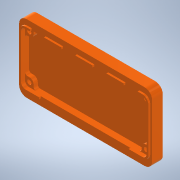
# Autodesk Inventor part: casing-bot
Saved by Autodesk Inventor 2021 (Build 250183000, 183)
## iProperties
Created: 2022-04-04
Part Number: casing-bot
Material: PET Plastic
Document SubType Name: Modeling
Designer: Staňa
Density: 1.541 g/cm^3
Appearance: Smooth - Light Orange
Author: Staňa
Autodesk Inventor part; units mm, degrees
ref_plane "YZ Plane" through (0, 0, 0) normal (1, 0, 0) x (0, 1, 0)
ref_plane "XZ Plane" through (0, 0, 0) normal (0, 1, 0) x (-1, 0, 0)
ref_plane "XY Plane" through (0, 0, 0) normal (0, 0, 1) x (1, 0, 0)
sketch "Sketch2" plane through (0, 0, 0) normal (0, 0, 1) x (1, 0, 0)
  line L0 (-50, -20) -> (-50, 15) construction
  arc A0 (-46.75, 18.25) -> (-50, 15) centre (-46.7497, 14.9997) ccw construction
  line L1 (-46.75, 18.25) -> (46.75, 18.25) construction
  arc A1 (50, 15) -> (46.75, 18.25) centre (46.7497, 14.9997) ccw construction
  line L2 (50, 15) -> (50, -20) construction
  arc A2 (46.75, -23.25) -> (50, -20) centre (46.7497, -19.9997) ccw construction
  line L3 (46.75, -23.25) -> (-46.75, -23.25) construction
  arc A3 (-50, -20) -> (-46.75, -23.25) centre (-46.7497, -19.9997) ccw construction
  circle A4 centre (-46.75, -22.184) radius 0.254 construction
  circle A5 centre (-48.934, -20) radius 0.254 construction
  circle A6 centre (-48.295, -21.545) radius 0.254 construction
  circle A7 centre (-45.205, -21.545) radius 0.254 construction
  circle A8 centre (-27.94, -19.9) radius 0.51 construction
  circle A9 centre (-44.566, -20) radius 0.254 construction
  circle A10 centre (-25.4, -19.9) radius 0.51 construction
  circle A11 centre (-48.295, -18.455) radius 0.254 construction
  circle A12 centre (-46.75, -20) radius 1.6 construction
  circle A13 centre (-46.75, -17.816) radius 0.254 construction
  circle A14 centre (-45.205, -18.455) radius 0.254 construction
  circle A15 centre (-30.48, -17.36) radius 0.51 construction
  circle A16 centre (-30.48, -19.9) radius 0.51 construction
  circle A17 centre (-27.94, -17.36) radius 0.51 construction
  circle A18 centre (-25.4, -17.36) radius 0.51 construction
  circle A19 centre (-17.78, -19.9) radius 0.51 construction
  circle A20 centre (-22.86, -19.9) radius 0.51 construction
  circle A21 centre (-20.32, -19.9) radius 0.51 construction
  circle A22 centre (-10.16, -19.9) radius 0.51 construction
  circle A23 centre (-7.62, -19.9) radius 0.51 construction
  circle A24 centre (-15.24, -19.9) radius 0.51 construction
  circle A25 centre (-12.7, -19.9) radius 0.51 construction
  circle A26 centre (-12.7, -17.36) radius 0.51 construction
  circle A27 centre (-5.08, -19.9) radius 0.51 construction
  circle A28 centre (-7.62, -17.36) radius 0.51 construction
  circle A29 centre (-5.08, -17.36) radius 0.51 construction
  circle A30 centre (-2.54, -19.9) radius 0.51 construction
  circle A31 centre (0, -19.9) radius 0.51 construction
  circle A32 centre (-2.54, -17.36) radius 0.51 construction
  circle A33 centre (0, -17.36) radius 0.51 construction
  circle A34 centre (-46.75, 12.816) radius 0.254 construction
  circle A35 centre (-48.295, 13.455) radius 0.254 construction
  circle A36 centre (-45.205, 13.455) radius 0.254 construction
  circle A37 centre (-41.31, 11.85) radius 0.51 construction
  circle A38 centre (-38.77, 11.85) radius 0.51 construction
  circle A39 centre (-41.31, 14.39) radius 0.51 construction
  circle A40 centre (-36.23, 11.85) radius 0.51 construction
  circle A41 centre (-48.934, 15) radius 0.254 construction
  circle A42 centre (-46.75, 15) radius 1.6 construction
  circle A43 centre (-48.295, 16.545) radius 0.254 construction
  circle A44 centre (-46.75, 17.184) radius 0.254 construction
  circle A45 centre (-38.77, 14.39) radius 0.51 construction
  circle A46 centre (-36.23, 14.39) radius 0.51 construction
  circle A47 centre (-45.205, 16.545) radius 0.254 construction
  circle A48 centre (-44.566, 15) radius 0.254 construction
  circle A49 centre (-20.32, -17.36) radius 0.51 construction
  circle A50 centre (-33.69, 11.85) radius 0.51 construction
  circle A51 centre (-22.86, -17.36) radius 0.51 construction
  circle A52 centre (-17.78, -17.36) radius 0.51 construction
  circle A53 centre (-15.24, -17.36) radius 0.51 construction
  circle A54 centre (-16.31, 11.85) radius 0.51 construction
  circle A55 centre (-10.16, -17.36) radius 0.51 construction
  circle A56 centre (-16.31, 14.39) radius 0.51 construction
  circle A57 centre (-13.77, 11.85) radius 0.51 construction
  circle A58 centre (-33.69, 14.39) radius 0.51 construction
  circle A59 centre (-13.77, 14.39) radius 0.51 construction
  circle A60 centre (-11.23, 11.85) radius 0.51 construction
  circle A61 centre (-8.69, 11.85) radius 0.51 construction
  circle A62 centre (-11.23, 14.39) radius 0.51 construction
  circle A63 centre (-8.69, 14.39) radius 0.51 construction
  circle A64 centre (10.16, -19.9) radius 0.51 construction
  circle A65 centre (5.08, -19.9) radius 0.51 construction
  circle A66 centre (7.62, -19.9) radius 0.51 construction
  circle A67 centre (20.32, -19.9) radius 0.51 construction
  circle A68 centre (22.86, -19.9) radius 0.51 construction
  circle A69 centre (12.7, -19.9) radius 0.51 construction
  circle A70 centre (15.24, -19.9) radius 0.51 construction
  circle A71 centre (2.54, -19.9) radius 0.51 construction
  circle A72 centre (7.62, -17.36) radius 0.51 construction
  circle A73 centre (10.16, -17.36) radius 0.51 construction
  circle A74 centre (12.7, -17.36) radius 0.51 construction
  circle A75 centre (15.24, -17.36) radius 0.51 construction
  circle A76 centre (17.78, -19.9) radius 0.51 construction
  circle A77 centre (17.78, -17.36) radius 0.51 construction
  circle A78 centre (20.32, -17.36) radius 0.51 construction
  circle A79 centre (25.4, -19.9) radius 0.51 construction
  circle A80 centre (30.48, -19.9) radius 0.51 construction
  circle A81 centre (44.566, -20) radius 0.254 construction
  circle A82 centre (45.205, -21.545) radius 0.254 construction
  circle A83 centre (46.75, -22.184) radius 0.254 construction
  circle A84 centre (48.295, -21.545) radius 0.254 construction
  circle A85 centre (48.934, -20) radius 0.254 construction
  circle A86 centre (22.86, -17.36) radius 0.51 construction
  circle A87 centre (27.94, -19.9) radius 0.51 construction
  circle A88 centre (25.4, -17.36) radius 0.51 construction
  circle A89 centre (27.94, -17.36) radius 0.51 construction
  circle A90 centre (45.205, -18.455) radius 0.254 construction
  circle A91 centre (46.75, -20) radius 1.6 construction
  circle A92 centre (46.75, -17.816) radius 0.254 construction
  circle A93 centre (48.295, -18.455) radius 0.254 construction
  circle A94 centre (2.54, -17.36) radius 0.51 construction
  circle A95 centre (0, 6.27) radius 0.5 construction
  circle A96 centre (0, 3.73) radius 0.5 construction
  circle A97 centre (5.08, -17.36) radius 0.51 construction
  circle A98 centre (30.48, -17.36) radius 0.51 construction
  circle A99 centre (8.69, 11.85) radius 0.51 construction
  circle A100 centre (11.23, 11.85) radius 0.51 construction
  circle A101 centre (8.69, 14.39) radius 0.51 construction
  circle A102 centre (13.77, 11.85) radius 0.51 construction
  circle A103 centre (11.23, 14.39) radius 0.51 construction
  circle A104 centre (13.77, 14.39) radius 0.51 construction
  circle A105 centre (16.31, 11.85) radius 0.51 construction
  circle A106 centre (33.69, 11.85) radius 0.51 construction
  circle A107 centre (16.31, 14.39) radius 0.51 construction
  circle A108 centre (33.69, 14.39) radius 0.51 construction
  circle A109 centre (36.23, 11.85) radius 0.51 construction
  circle A110 centre (38.77, 11.85) radius 0.51 construction
  circle A111 centre (41.31, 14.39) radius 0.51 construction
  circle A112 centre (41.31, 11.85) radius 0.51 construction
  circle A113 centre (46.75, 12.816) radius 0.254 construction
  circle A114 centre (45.205, 13.455) radius 0.254 construction
  circle A115 centre (48.295, 13.455) radius 0.254 construction
  circle A116 centre (36.23, 14.39) radius 0.51 construction
  circle A117 centre (38.77, 14.39) radius 0.51 construction
  circle A118 centre (44.566, 15) radius 0.254 construction
  circle A119 centre (45.205, 16.545) radius 0.254 construction
  circle A120 centre (46.75, 15) radius 1.6 construction
  circle A121 centre (48.934, 15) radius 0.254 construction
  circle A122 centre (46.75, 17.184) radius 0.254 construction
  circle A123 centre (48.295, 16.545) radius 0.254 construction
  line L4 (-46.7497, -23.5) -> (46.7497, -23.5)
  arc A124 (46.7497, -23.5) -> (50.25, -19.9997) centre (46.7497, -19.9997) ccw
  line L5 (50.25, -19.9997) -> (50.25, 14.9997)
  arc A125 (50.25, 14.9997) -> (46.7497, 18.5) centre (46.7497, 14.9997) ccw
  line L6 (46.7497, 18.5) -> (-46.7497, 18.5)
  arc A126 (-46.7497, 18.5) -> (-50.25, 14.9997) centre (-46.7497, 14.9997) ccw
  line L7 (-50.25, 14.9997) -> (-50.25, -19.9997)
  arc A127 (-50.25, -19.9997) -> (-46.7497, -23.5) centre (-46.7497, -19.9997) ccw
  line L8 (-32.1701, 24.2499) -> (-42.8301, 24.2499) construction
  line L9 (34.9801, -30.2999) -> (-34.9799, -30.2999) construction
  line L10 (-53.25, 18.2499) -> (-53.25, -24.2999)
  line L11 (53.25, -24.2999) -> (53.25, 18.2499)
  line L12 (-47.25, -30.2999) -> (47.25, -30.2999)
  line L13 (47.25, 24.2499) -> (-47.25, 24.2499)
  arc A128 (-53.25, -24.2999) -> (-47.25, -30.2999) centre (-47.25, -24.2999) ccw
  arc A129 (-47.25, 24.2499) -> (-53.25, 18.2499) centre (-47.25, 18.2499) ccw
  arc A130 (53.25, 18.2499) -> (47.25, 24.2499) centre (47.25, 18.2499) ccw
  arc A131 (47.25, -30.2999) -> (53.25, -24.2999) centre (47.25, -24.2999) ccw
  point P0 (0, 0)
  dimension "d4" = 0.25
  dimension "d7" = 3
  dimension "d8" = 3
  dimension "d10" = 6
  constraints: 16 end point, 16 point on circle, 8 centre point, 8 tangent, 3 equal radius, 2 collinear, 2 parallel, 7 other
  measures "d4" radial gap between concentric circles of A3 A127
  measures "d7" distance between parallel lines of L7 L10
  measures "d8" distance between parallel lines of L5 L11
  measures "d10" radius of A128
extrude "Extrusion1" add sketch "Sketch2" against normal blind 5
sketch "Sketch6" plane through (0, 0, 0) normal (0, 0, 1) x (1, 0, 0)
  line L0 (-50.25, -19.9997) -> (-50.25, 14.9997) projected
  arc A0 (-50.25, -19.9997) -> (-46.7497, -23.5) centre (-46.7497, -19.9997) ccw projected
  line L1 (46.7497, -23.5) -> (-46.7497, -23.5) projected
  arc A1 (46.7497, -23.5) -> (50.25, -19.9997) centre (46.7497, -19.9997) ccw projected
  line L2 (50.25, 14.9997) -> (50.25, -19.9997) projected
  arc A2 (50.25, 14.9997) -> (46.7497, 18.5) centre (46.7497, 14.9997) ccw projected
  line L3 (-46.7497, 18.5) -> (46.7497, 18.5) projected
  arc A3 (-46.7497, 18.5) -> (-50.25, 14.9997) centre (-46.7497, 14.9997) ccw projected
  line L4 (-42.8301, 24.2499) -> (-42.8301, 15.7499) construction
  line L5 (-32.1701, 15.7499) -> (-32.1701, 24.2499) construction
  line L6 (-17.8301, 24.2499) -> (-17.8301, 15.7499) construction
  line L7 (-7.1701, 15.7499) -> (-7.1701, 24.2499) construction
  line L8 (7.1699, 24.2499) -> (7.1699, 15.7499) construction
  line L9 (17.8299, 15.7499) -> (17.8299, 24.2499) construction
  line L10 (32.1699, 24.2499) -> (32.1699, 15.7499) construction
  line L11 (42.8299, 15.7499) -> (42.8299, 24.2499) construction
  line L12 (35.5801, -21.4999) -> (35.5801, -30.2999) construction
  line L13 (-35.5799, -30.2999) -> (-35.5799, -21.4999) construction
  line L14 (-51.75, 14.9997) -> (-51.75, -19.9997)
  arc A4 (-51.75, -19.9997) -> (-46.7497, -25) centre (-46.7497, -19.9997) ccw
  line L15 (-46.7497, -25) -> (-35.8299, -25)
  arc A5 (46.7497, -25) -> (51.75, -19.9997) centre (46.7497, -19.9997) ccw
  line L16 (51.75, -19.9997) -> (51.75, 14.9997)
  arc A6 (51.75, 14.9997) -> (46.7497, 20) centre (46.7497, 14.9997) ccw
  line L17 (46.7497, 20) -> (-46.7497, 20)
  arc A7 (-46.7497, 20) -> (-51.75, 14.9997) centre (-46.7497, 14.9997) ccw
  line L18 (-35.8299, -25) -> (-35.8299, -23.5)
  line L19 (35.8301, -23.5) -> (35.8301, -25)
  line L20 (35.8301, -25) -> (46.7497, -25)
  line L21 (-43.0801, 20) -> (-43.0801, 18.5)
  line L22 (-31.9201, 18.5) -> (-31.9201, 20)
  line L23 (-18.0801, 20) -> (-18.0801, 18.5)
  line L24 (-6.9201, 18.5) -> (-6.9201, 20)
  line L25 (6.9199, 20) -> (6.9199, 18.5)
  line L26 (18.0799, 18.5) -> (18.0799, 20)
  line L27 (31.9199, 20) -> (31.9199, 18.5)
  line L28 (43.0799, 18.5) -> (43.0799, 20)
  point P0 (0, 0)
  dimension "d18" = 1.5
  dimension "d19" = 0.25
  dimension "d20" = 0.25
  dimension "d21" = 0.25
  dimension "d22" = 0.25
  dimension "d23" = 0.25
  dimension "d24" = 0.25
  dimension "d25" = 0.25
  dimension "d26" = 0.25
  dimension "d27" = 0.25
  dimension "d28" = 0.25
  constraints: 28 end point, 10 parallel, 8 point on circle, 4 centre point, 3 tangent, 2 concentric, 2 perpendicular, 2 point on line, 23 other
  measures "d18" distance between parallel lines of L0 L14
  measures "d19" distance between parallel lines of L13 L18
  measures "d20" distance between parallel lines of L12 L19
  measures "d21" distance between parallel lines of L4 L21
  measures "d22" distance between parallel lines of L5 L22
  measures "d23" distance between parallel lines of L6 L23
  measures "d24" distance between parallel lines of L7 L24
  measures "d25" distance between parallel lines of L8 L25
  measures "d26" distance between parallel lines of L9 L26
  measures "d27" distance between parallel lines of L10 L27
  measures "d28" distance between parallel lines of L11 L28
extrude "Extrusion4" add sketch "Sketch6" along normal blind 1.5 contours A0 L1 L18 L15 A4 L14 A7 L17 L21 L3 A3 L0 | L1 A1 L2 A2 L3 L28 L17 A6 L16 A5 L20 L19 | L22 L17 L23 L3 | L24 L17 L25 L3 | L26 L17 L27 L3
sketch "Sketch5" plane through (0, 0, -5) normal (0, 0, -1) x (-1, 0, 0)
  arc A0 (47.25, -30.2999) -> (53.25, -24.2999) centre (47.25, -24.2999) ccw projected
  line L0 (-47.25, -30.2999) -> (47.25, -30.2999) projected
  line L1 (53.25, -24.2999) -> (53.25, 18.2499) projected
  arc A1 (53.25, 18.2499) -> (47.25, 24.2499) centre (47.25, 18.2499) ccw projected
  line L2 (47.25, 24.2499) -> (-47.25, 24.2499) projected
  arc A2 (-47.25, 24.2499) -> (-53.25, 18.2499) centre (-47.25, 18.2499) ccw projected
  line L3 (-53.25, 18.2499) -> (-53.25, -24.2999) projected
  arc A3 (-53.25, -24.2999) -> (-47.25, -30.2999) centre (-47.25, -24.2999) ccw projected
  point P0 (0, 0)
extrude "Extrusion3" add sketch "Sketch5" along normal blind 3.5
sketch "Sketch7" plane through (0, 0, -5) normal (0, 0, 1) x (1, 0, 0)
  circle A0 centre (-46.75, 15) radius 1.6 construction
  circle A1 centre (-46.75, -20) radius 1.6 construction
  circle A2 centre (46.75, -20) radius 1.6 construction
  circle A3 centre (46.75, 15) radius 1.6 construction
  line L0 (-50.25, 14.9997) -> (-50.25, -19.9997) projected
  arc A4 (-50.25, -19.9997) -> (-46.7497, -23.5) centre (-46.7497, -19.9997) ccw projected
  line L1 (-46.7497, -23.5) -> (46.7497, -23.5) projected
  arc A5 (46.7497, -23.5) -> (50.25, -19.9997) centre (46.7497, -19.9997) ccw projected
  line L2 (50.25, -19.9997) -> (50.25, 14.9997) projected
  arc A6 (50.25, 14.9997) -> (46.7497, 18.5) centre (46.7497, 14.9997) ccw projected
  line L3 (46.7497, 18.5) -> (-46.7497, 18.5) projected
  arc A7 (-46.7497, 18.5) -> (-50.25, 14.9997) centre (-46.7497, 14.9997) ccw projected
  arc A8 (43.2497, 14.9997) -> (46.7497, 11.4997) centre (46.7497, 14.9997) ccw
  line L4 (46.7497, 11.4997) -> (48.2497, 11.4997)
  line L5 (43.2497, 14.9997) -> (43.2497, 16.4997)
  line L6 (50.25, -19.9997) -> (50.25, 14.9997) projected
  arc A9 (50.25, 9.4993) -> (48.2497, 11.4997) centre (48.2497, 9.4993) ccw
  line L7 (46.7497, 18.5) -> (-46.7497, 18.5) projected
  arc A10 (43.2497, 16.4997) -> (41.2493, 18.5) centre (41.2493, 16.4997) ccw
  line L8 (0, 40.6706) -> (0, -44.651) construction
  arc A11 (-46.7497, 11.4997) -> (-43.2497, 14.9997) centre (-46.7497, 14.9997) ccw
  line L9 (-46.7497, 11.4997) -> (-48.2497, 11.4997)
  line L10 (-43.2497, 14.9997) -> (-43.2497, 16.4997)
  arc A12 (-48.2497, 11.4997) -> (-50.25, 9.4993) centre (-48.2497, 9.4993) ccw
  arc A13 (-41.2493, 18.5) -> (-43.2497, 16.4997) centre (-41.2493, 16.4997) ccw
  arc A14 (46.7497, -16.4997) -> (43.2497, -19.9997) centre (46.7497, -19.9997) ccw
  line L11 (46.7497, -16.4997) -> (48.2497, -16.4997)
  line L12 (43.2497, -19.9997) -> (43.2497, -21.4997)
  arc A15 (48.2497, -16.4997) -> (50.25, -14.4993) centre (48.2497, -14.4993) ccw
  line L13 (-46.7497, -23.5) -> (46.7497, -23.5) projected
  arc A16 (41.2493, -23.5) -> (43.2497, -21.4997) centre (41.2493, -21.4997) ccw
  arc A17 (-43.2497, -19.9997) -> (-46.7497, -16.4997) centre (-46.7497, -19.9997) ccw
  line L14 (-46.7497, -16.4997) -> (-48.2497, -16.4997)
  line L15 (-43.2497, -19.9997) -> (-43.2497, -21.4997)
  arc A18 (-50.25, -14.4993) -> (-48.2497, -16.4997) centre (-48.2497, -14.4993) ccw
  arc A19 (-43.2497, -21.4997) -> (-41.2493, -23.5) centre (-41.2493, -21.4997) ccw
  point P0 (0, 0)
  point P1 (50.25, -14.9993)
  point P2 (40.7493, -23.5)
  point P3 (41.7493, 18.5)
  point P4 (50.25, 9.4993)
  point P5 (-40.7493, -23.5)
  point P6 (-50.25, -14.9993)
  point P7 (-50.25, 9.4993)
  point P8 (-41.7493, 18.5)
  point P9 (50.25, -13.9993)
  point P10 (-50.25, -13.9993)
  point P11 (-40.7493, -23.5)
  point P12 (-41.7493, 18.5)
  point P13 (-41.7493, -23.5)
  point P14 (50.25, -14.4993)
  point P15 (-50.25, -14.4993)
  point P16 (-41.2493, -23.5)
  point P17 (-41.2493, 18.5)
  dimension "d31" = 3.5
  dimension "d32" = 1.5
  constraints: 24 point on circle, 18 end point, 18 symmetric about line, 12 centre point, 9 tangent, 5 point on line, 4 equal radius, 3 equal length, 3 vertical, 2 coincident, 2 horizontal, 6 other
  measures "d31" radius of A8
  measures "d32" distance of L4.start L4.end
ref_plane "Work Plane2" through (-50, -23.25, -1.6) normal (0, 0, -1) x (0, 1, 0)
extrude "Extrusion5" add sketch "Sketch7" along normal up to surface (3.4 mm away) contours A7 L3 A13 L10 A11 L9 A12 L0 | A18 L14 A17 L15 A19 L1 A4 L0 | L3 A6 L2 A9 L4 A8 L5 A10 | A16 L12 A14 L11 A15 L2 A5 L1
sketch "Sketch8" plane through (0, 0, -8.5) normal (0, 0, -1) x (-1, 0, 0)
  circle A0 centre (46.75, -20) radius 1.6 construction
  circle A1 centre (46.75, 15) radius 1.6 construction
  circle A2 centre (-46.75, 15) radius 1.6 construction
  circle A3 centre (-46.75, -20) radius 1.6 construction
  point P0 (0, 0)
hole "Hole2" at (-46.75, -20, -8.5) at (-46.75, 15, -8.5) at (46.75, 15, -8.5) at (46.75, -20, -8.5) direction (0, 0, 1) diameter 3.4 end through all counterbore diameter 5.7 counterbore depth 2.2 clearance for "Hex Head Cap Screw ISO 24017" size "M3" standard "ISO"
equation "\"d8\" = d7"
equation "\"d20\" = d19"
equation "\"d21\" = d19"
equation "\"d22\" = d19"
equation "\"d23\" = d19"
equation "\"d24\" = d19"
equation "\"d25\" = d19"
equation "\"d26\" = d19"
equation "\"d27\" = d19"
equation "\"d28\" = d19"
body "Solid1"
